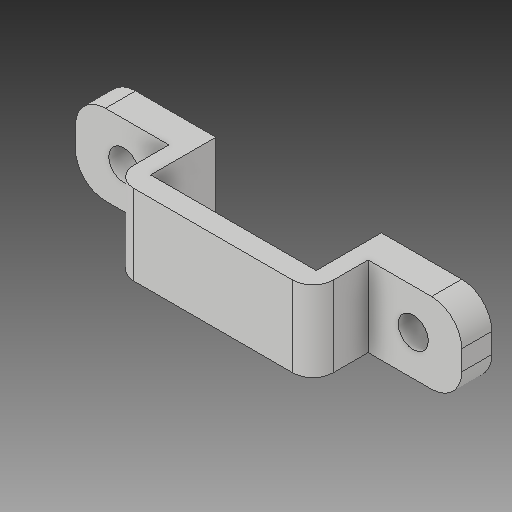
# Autodesk Inventor part: Smaller ethernet holder
Saved by Autodesk Inventor 2018 (Build 220112000, 112)
## iProperties
Created: 2019-10-18
Part Number: Smaller ethernet holder
Material: Generic
Document SubType Name: Modeling
Designer: Jacob
Density: 1 g/cm^3
Appearance: Default
Mass: 0.860077 g
Surface Area: 10.7105 cm^2
Volume: 0.860077 cm^3
Author: Jacob
Autodesk Inventor part; units mm, degrees
ref_plane "YZ Plane" through (0, 0, 0) normal (1, 0, 0) x (0, 1, 0)
ref_plane "XZ Plane" through (0, 0, 0) normal (0, 1, 0) x (-1, 0, 0)
ref_plane "XY Plane" through (0, 0, 0) normal (0, 0, 1) x (1, 0, 0)
sketch "Sketch1" plane through (0, 0, 0) normal (0, 0, 1) x (1, 0, 0)
  line L0 (-8.25, 4) -> (8.25, 4)
  line L1 (8.25, 4) -> (8.25, -4)
  line L2 (8.25, -4) -> (-8.25, -4)
  line L3 (-8.25, -4) -> (-8.25, 4)
  line L4 (-8.25, 4) -> (8.25, -4) construction
  line L5 (8.25, 4) -> (-8.25, -4) construction
  point P0 (0, 0)
  dimension "d0" = 8
  dimension "d1" = 16.5
  constraints: 12 end point, 2 midpoint, 2 parallel, 1 horizontal, 1 perpendicular
  measures "d0" distance between parallel lines of L2 L0
  measures "d1" distance of L0.start L0.end
extrude "Extrusion1" add sketch "Sketch1" along normal blind 6.5
shell "Shell1" thickness 3 outward yes removed faces 3 at (-2.75, 4, 2.1667) at (-2.75, -1.3333, 0) at (2.75, -4, 2.1667)
sketch "Sketch2" plane through (0, 0, 0) normal (0, 0, -1) x (-1, 0, 0)
  line L0 (0, 0) -> (24.1853, 0) construction
  line L1 (0, 0) -> (-21.4018, 0) construction
  line L2 (-19.25, 4) -> (-11.25, 4)
  line L3 (-11.25, 4) -> (-11.25, -4)
  line L4 (-11.25, -4) -> (-19.25, -4)
  line L5 (-19.25, -4) -> (-19.25, 4)
  line L6 (-19.25, 4) -> (-11.25, -4) construction
  line L7 (-11.25, 4) -> (-19.25, -4) construction
  line L8 (11.25, 4) -> (19.25, 4)
  line L9 (19.25, 4) -> (19.25, -4)
  line L10 (19.25, -4) -> (11.25, -4)
  line L11 (11.25, -4) -> (11.25, 4)
  line L12 (11.25, 4) -> (19.25, -4) construction
  line L13 (19.25, 4) -> (11.25, -4) construction
  line L14 (-11.25, 4) -> (-11.25, -4) projected
  line L15 (11.25, -4) -> (11.25, 4) projected
  point P0 (-15.25, 0)
  point P1 (15.25, 0)
  dimension "d5" = 0
  dimension "d6" = 8
  dimension "d7" = 8
  dimension "d8" = 0
  dimension "d9" = 8
  dimension "d10" = 8
  constraints: 28 end point, 4 horizontal, 4 midpoint, 4 parallel, 2 perpendicular, 2 point on line
  measures "d5" distance between parallel lines of L14 L3
  measures "d6" distance of L2.start L2.end
  measures "d7" distance of L4.end L2.start
  measures "d8" distance between parallel lines of L15 L11
  measures "d9" distance of L8.start L8.end
  measures "d10" distance of L8.end L9.end
extrude "Extrusion2" add sketch "Sketch2" against normal blind 3
sketch "Sketch3" plane through (0, 0, 0) normal (0, 0, -1) x (-1, 0, 0)
  line L0 (-19.25, -4) -> (-19.25, 4) projected
  line L1 (-19.25, 0) -> (17.977, 0) construction
  line L2 (-11.25, 4) -> (11.25, 4) projected
  line L3 (0, 4) -> (0, -4) construction
  line L4 (8.25, -4) -> (-8.25, -4) projected
  circle A0 centre (-14.425, 0) radius 1.5
  circle A1 centre (14.425, 0) radius 1.5
  point P0 (0, 0)
  dimension "d13" = 28.85
  dimension "d14" = 14.425
  dimension "d15" = 14.425
  dimension "d16" = 3
  dimension "d17" = 3
  constraints: 4 end point, 3 midpoint, 2 centre point, 2 point on line, 1 horizontal
  measures "d13" distance of A1.centre A0.centre
  measures "d14" distance from line of L3 A0.centre
  measures "d15" distance from line of L3 A1.centre
  measures "d16" diameter of A0
  measures "d17" diameter of A1
extrude "Extrusion3" cut sketch "Sketch3" against normal blind 5
fillet "Fillet1" radius 3 4 edges at (19.25, 4, 1.5) (19.25, -4, 1.5) (-19.25, 4, 1.5) (-19.25, -4, 1.5)
sketch "Sketch4" plane through (0, 0, 3) normal (0, 0, 1) x (1, 0, 0)
  line L0 (-18.925, 4) -> (-9.925, 4)
  line L1 (-9.925, 4) -> (-9.925, -4)
  line L2 (-9.925, -4) -> (-18.925, -4)
  line L3 (-18.925, -4) -> (-18.925, 4)
  circle A0 centre (-14.425, 0) radius 1.5 projected
  line L4 (-18.925, 4) -> (-9.925, -4) construction
  line L5 (-9.925, 4) -> (-18.925, -4) construction
  line L6 (9.925, 4) -> (18.925, 4)
  line L7 (18.925, 4) -> (18.925, -4)
  line L8 (18.925, -4) -> (9.925, -4)
  line L9 (9.925, -4) -> (9.925, 4)
  circle A1 centre (14.425, 0) radius 1.5 projected
  line L10 (9.925, 4) -> (18.925, -4) construction
  line L11 (18.925, 4) -> (9.925, -4) construction
  point P0 (0, 0)
  dimension "d25" = 9
  dimension "d26" = 8
  dimension "d27" = 8
  dimension "d28" = 9
  constraints: 24 end point, 4 midpoint, 4 parallel, 2 horizontal, 2 perpendicular
  measures "d25" distance of L0.start L0.end
  measures "d26" distance of L2.end L0.start
  measures "d27" distance of L6.end L7.end
  measures "d28" distance of L6.start L6.end
extrude "Extrusion4" cut sketch "Sketch4" along normal blind 25.4
sketch "Sketch6" plane through (0, 0, 9.5) normal (0, 0, 1) x (1, 0, 0)
  line L0 (-9.925, 4) -> (-9.925, -4) projected
  line L1 (9.925, -4) -> (9.925, 4) projected
  line L2 (-9.925, 4) -> (9.925, 4)
  line L3 (9.925, 4) -> (9.925, -4)
  line L4 (9.925, -4) -> (-9.925, -4)
  line L5 (-9.925, -4) -> (-9.925, 4)
  point P0 (0, 0)
  constraints: 8 end point, 2 parallel, 1 horizontal, 1 perpendicular
extrude "Extrusion6" cut sketch "Sketch6" against normal blind 1
fillet "Fillet3" radius 2 2 edges at (-9.925, 0, 8.5) (9.925, 0, 8.5)
equation "\"d14\" = d15"
body "Solid1"
